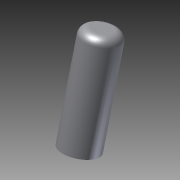
# Autodesk Inventor part: G-actuator
Saved by Autodesk Inventor 2011 SP1 (Build 150282100, 282)
## iProperties
Created: 2013-12-24
Part Number: G-actuator
Catalog Web Link: www.cadenas.de
Description: G Series - Process Sealed Ultra-Miniature Toggles -actuator-
Vendor: NKKSWITCHES
Document SubType Name: Modeling
Designer: PARTuser1
Manufacturer: NKKSWITCHES
Density: 1 g/cm^3
Category: PARTsolutions
Company: NKKSWITCHES
Title: G-actuator
Author: Cadenas PARTsolutions
PSOL_IDENT_0: {$CADENAS_DATA\23d-libs\nkkswitches\toggle\g\parts\g_actuator.prj},215 {VTYP=3D},{NB=G-actuator},{LI
PSOL_IDENT_1: NA=G-actuator},{NN=G Series - Process Sealed Ultra-Miniature Toggles -actuator},{DATE=12.03.2009 08:
PSOL_IDENT_2: 26:50},{GEOMDATE=12.03.2009 00:00:00},{VERSION=},{LINEID=10},{LINESUBID=-1},{WBVAR=}  {NB=G-actuator
PSOL_IDENT_3: },{LINA=G-actuator},{KT=DUMMY},{PN=G},{SRS=G}
CNS_NN: G Series - Process Sealed Ultra-Miniature Toggles -actuator
CNS_NB: G-actuator
CNS_NBSYN: $PN.-actuator
CNS_LINA: G-actuator
CNS_PN: G
CNS_SRS: G
SUPPLIER: NKKSWITCHES
ARTICLENO: G-actuator
BOMINFO: G-actuator
CREATOR: CADENAS GmbH
Autodesk Inventor part; units mm, degrees
sketch "Sketch_1" plane through (0, 0, 0) normal (1, 0, 0) x (0, 1, 0)
  line L0 (0.635, 0) -> (5.2684, -1.1552)
  line L1 (5.2684, -1.1552) -> (5.1547, -1.6112)
  arc A0 (4.6928, -1.8887) -> (5.1547, -1.6112) centre (4.785, -1.519) ccw
  line L2 (4.6928, -1.8887) -> (0.4291, -0.8256)
  line L3 (0.4291, -0.8256) -> (0.635, 0)
  line L4 (0.635, 0) -> (5.2684, -1.1552)
  constraints: 10 end point, 2 point on circle, 1 centre point
revolve "Revolution1" add sketch "Sketch_1" angle 360 about axis through (0, 0.635, 0) along (0, -0.9702957, 0.2419219)
ref_plane "to_body_XY" through (0, 0, 0) normal (0, 1, 0) x (1, 0, 0)
ref_plane "to_body_YZ" through (0, 0, 0) normal (1, 0, 0) x (0, 0, -1)
ref_plane "to_body_ZX" through (0, 0, 0) normal (0, 0, -1) x (0, 1, 0)
body "Solid1"
